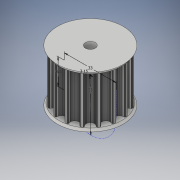
# Autodesk Inventor part: 8M_pulley_39mm
Saved by Autodesk Inventor 2019 (Build 230136000, 136)
## iProperties
Created: 2019-09-25
Part Number: 8M_pulley_39mm
Material: Generic
Document SubType Name: Modeling
Designer: isaac
Density: 1 g/cm^3
Appearance: Default
Author: isaac
Autodesk Inventor part; units mm, degrees
(part 1 of 2)
sketch "Sketch1" plane through (0, 0, 0) normal (0, 1, 0) x (-1, 0, 0)
  line L0 (-19.3836, -3.3292) -> (-19.3679, -3.8461)
  line L1 (-19.3679, -3.8461) -> (-19.3017, -4.359)
  line L2 (-19.3017, -4.359) -> (-19.3017, -4.3591)
  line L3 (-19.3017, -4.3591) -> (-19.2707, -4.4187)
  line L4 (-19.2707, -4.4187) -> (-19.1879, -4.5272)
  line L5 (-19.1879, -4.5272) -> (-19.0895, -4.6186)
  line L6 (-19.0895, -4.6186) -> (-18.9784, -4.6913)
  line L7 (-18.9784, -4.6913) -> (-18.8571, -4.7439)
  line L8 (-18.8571, -4.7439) -> (-18.7285, -4.775)
  line L9 (-18.7285, -4.775) -> (-18.5953, -4.7829)
  line L10 (-18.5953, -4.7829) -> (-18.4601, -4.7664)
  line L11 (-18.4601, -4.7664) -> (-17.6457, -4.5321)
  line L12 (-17.6457, -4.5321) -> (-17.4212, -4.494)
  line L13 (-17.4212, -4.494) -> (-17.1971, -4.4763)
  line L14 (-17.1971, -4.4763) -> (-16.9744, -4.4785)
  line L15 (-16.9744, -4.4785) -> (-16.7542, -4.4999)
  line L16 (-16.7542, -4.4999) -> (-16.5375, -4.5401)
  line L17 (-16.5375, -4.5401) -> (-16.3256, -4.5984)
  line L18 (-16.3256, -4.5984) -> (-16.1194, -4.6743)
  line L19 (-16.1194, -4.6743) -> (-15.92, -4.7673)
  line L20 (-15.92, -4.7673) -> (-15.7285, -4.8767)
  line L21 (-15.7285, -4.8767) -> (-15.5461, -5.0021)
  line L22 (-15.5461, -5.0021) -> (-15.3737, -5.1428)
  line L23 (-15.3737, -5.1428) -> (-15.2125, -5.2982)
  line L24 (-15.2125, -5.2982) -> (-15.0635, -5.4679)
  line L25 (-15.0635, -5.4679) -> (-14.9279, -5.6513)
  line L26 (-14.9279, -5.6513) -> (-14.8067, -5.8478)
  line L27 (-14.8067, -5.8478) -> (-14.7009, -6.0568)
  line L28 (-14.7009, -6.0568) -> (-14.6281, -6.2792)
  line L29 (-14.6281, -6.2792) -> (-14.575, -6.5038)
  line L30 (-14.575, -6.5038) -> (-14.5414, -6.7293)
  line L31 (-14.5414, -6.7293) -> (-14.5268, -6.9545)
  line L32 (-14.5268, -6.9545) -> (-14.5309, -7.1784)
  line L33 (-14.5309, -7.1784) -> (-14.5534, -7.3996)
  line L34 (-14.5534, -7.3996) -> (-14.5938, -7.6172)
  line L35 (-14.5938, -7.6172) -> (-14.6518, -7.8299)
  line L36 (-14.6518, -7.8299) -> (-14.7271, -8.0366)
  line L37 (-14.7271, -8.0366) -> (-14.8192, -8.2361)
  line L38 (-14.8192, -8.2361) -> (-14.9278, -8.4272)
  line L39 (-14.9278, -8.4272) -> (-15.0525, -8.6088)
  line L40 (-15.0525, -8.6088) -> (-15.193, -8.7797)
  line L41 (-15.193, -8.7797) -> (-15.3488, -8.9388)
  line L42 (-15.3488, -8.9388) -> (-15.5197, -9.0849)
  line L43 (-15.5197, -9.0849) -> (-15.7052, -9.2168)
  line L44 (-15.7052, -9.2168) -> (-16.4468, -9.627)
  line L45 (-16.4468, -9.627) -> (-16.554, -9.711)
  line L46 (-16.554, -9.711) -> (-16.6426, -9.8109)
  line L47 (-16.6426, -9.8109) -> (-16.7116, -9.9238)
  line L48 (-16.7116, -9.9238) -> (-16.7601, -10.0467)
  line L49 (-16.7601, -10.0467) -> (-16.7873, -10.1767)
  line L50 (-16.7873, -10.1767) -> (-16.7923, -10.3108)
  line L51 (-16.7923, -10.3108) -> (-16.7741, -10.4461)
  line L52 (-16.7741, -10.4461) -> (-16.7538, -10.5101)
  line L53 (-16.7538, -10.5101) -> (-16.7538, -10.5102)
  line L54 (-16.7538, -10.5102) -> (-16.4879, -10.9538)
  line L55 (-16.4879, -10.9538) -> (-16.1799, -11.3692)
  line L56 (-16.1799, -11.3692) -> (-16.1653, -11.3814)
  line L57 (-16.1653, -11.3814) -> (-16.1652, -11.3814)
  line L58 (-16.1652, -11.3814) -> (-16.1284, -11.4124)
  line L59 (-16.1284, -11.4124) -> (-16.0103, -11.481)
  line L60 (-16.0103, -11.481) -> (-15.8845, -11.5278)
  line L61 (-15.8845, -11.5278) -> (-15.754, -11.5524)
  line L62 (-15.754, -11.5524) -> (-15.6218, -11.5546)
  line L63 (-15.6218, -11.5546) -> (-15.4911, -11.5341)
  line L64 (-15.4911, -11.5341) -> (-15.365, -11.4905)
  line L65 (-15.365, -11.4905) -> (-15.2464, -11.4235)
  line L66 (-15.2464, -11.4235) -> (-14.5837, -10.8953)
  line L67 (-14.5837, -10.8953) -> (-14.3909, -10.7742)
  line L68 (-14.3909, -10.7742) -> (-14.1905, -10.6721)
  line L69 (-14.1905, -10.6721) -> (-13.984, -10.5889)
  line L70 (-13.984, -10.5889) -> (-13.7723, -10.5244)
  line L71 (-13.7723, -10.5244) -> (-13.5568, -10.4787)
  line L72 (-13.5568, -10.4787) -> (-13.3387, -10.4514)
  line L73 (-13.3387, -10.4514) -> (-13.1191, -10.4426)
  line L74 (-13.1191, -10.4426) -> (-12.8993, -10.4522)
  line L75 (-12.8993, -10.4522) -> (-12.6806, -10.4801)
  line L76 (-12.6806, -10.4801) -> (-12.464, -10.526)
  line L77 (-12.464, -10.526) -> (-12.2509, -10.5901)
  line L78 (-12.2509, -10.5901) -> (-12.0425, -10.672)
  line L79 (-12.0425, -10.672) -> (-11.8399, -10.7718)
  line L80 (-11.8399, -10.7718) -> (-11.6444, -10.8893)
  line L81 (-11.6444, -10.8893) -> (-11.4572, -11.0244)
  line L82 (-11.4572, -11.0244) -> (-11.2796, -11.177)
  line L83 (-11.2796, -11.177) -> (-11.1271, -11.3547)
  line L84 (-11.1271, -11.3547) -> (-10.9922, -11.5418)
  line L85 (-10.9922, -11.5418) -> (-10.8748, -11.7373)
  line L86 (-10.8748, -11.7373) -> (-10.7752, -11.9398)
  line L87 (-10.7752, -11.9398) -> (-10.6933, -12.1481)
  line L88 (-10.6933, -12.1481) -> (-10.6293, -12.3611)
  line L89 (-10.6293, -12.3611) -> (-10.5834, -12.5776)
  line L90 (-10.5834, -12.5776) -> (-10.5556, -12.7963)
  line L91 (-10.5556, -12.7963) -> (-10.546, -13.0161)
  line L92 (-10.546, -13.0161) -> (-10.5548, -13.2356)
  line L93 (-10.5548, -13.2356) -> (-10.582, -13.4537)
  line L94 (-10.582, -13.4537) -> (-10.6278, -13.6692)
  line L95 (-10.6278, -13.6692) -> (-10.6921, -13.8809)
  line L96 (-10.6921, -13.8809) -> (-10.7753, -14.0875)
  line L97 (-10.7753, -14.0875) -> (-10.8772, -14.2879)
  line L98 (-10.8772, -14.2879) -> (-10.9981, -14.4808)
  line L99 (-10.9981, -14.4808) -> (-11.5263, -15.1435)
  line L100 (-11.5263, -15.1435) -> (-11.5932, -15.2621)
  line L101 (-11.5932, -15.2621) -> (-11.6368, -15.3883)
  line L102 (-11.6368, -15.3883) -> (-11.6573, -15.519)
  line L103 (-11.6573, -15.519) -> (-11.6551, -15.6512)
  line L104 (-11.6551, -15.6512) -> (-11.6305, -15.7817)
  line L105 (-11.6305, -15.7817) -> (-11.5838, -15.9075)
  line L106 (-11.5838, -15.9075) -> (-11.5152, -16.0255)
  line L107 (-11.5152, -16.0255) -> (-11.472, -16.0769)
  line L108 (-11.472, -16.0769) -> (-11.472, -16.077)
  line L109 (-11.472, -16.077) -> (-11.0566, -16.385)
  line L110 (-11.0566, -16.385) -> (-10.613, -16.6509)
  line L111 (-10.613, -16.6509) -> (-10.5948, -16.6567)
  line L112 (-10.5948, -16.6567) -> (-10.5489, -16.6712)
  line L113 (-10.5489, -16.6712) -> (-10.4136, -16.6894)
  line L114 (-10.4136, -16.6894) -> (-10.2794, -16.6844)
  line L115 (-10.2794, -16.6844) -> (-10.1494, -16.6572)
  line L116 (-10.1494, -16.6572) -> (-10.0264, -16.6087)
  line L117 (-10.0264, -16.6087) -> (-9.9135, -16.5397)
  line L118 (-9.9135, -16.5397) -> (-9.8137, -16.4511)
  line L119 (-9.8137, -16.4511) -> (-9.7298, -16.3439)
  line L120 (-9.7298, -16.3439) -> (-9.3196, -15.6022)
  line L121 (-9.3196, -15.6022) -> (-9.1879, -15.4166)
  line L122 (-9.1879, -15.4166) -> (-9.0419, -15.2456)
  line L123 (-9.0419, -15.2456) -> (-8.8829, -15.0896)
  line L124 (-8.8829, -15.0896) -> (-8.7121, -14.9491)
  line L125 (-8.7121, -14.9491) -> (-8.5305, -14.8243)
  line L126 (-8.5305, -14.8243) -> (-8.3394, -14.7156)
  line L127 (-8.3394, -14.7156) -> (-8.1399, -14.6235)
  line L128 (-8.1399, -14.6235) -> (-7.9332, -14.5482)
  line L129 (-7.9332, -14.5482) -> (-7.7204, -14.4902)
  line L130 (-7.7204, -14.4902) -> (-7.5028, -14.4498)
  line L131 (-7.5028, -14.4498) -> (-7.2814, -14.4274)
  line L132 (-7.2814, -14.4274) -> (-7.0575, -14.4233)
  line L133 (-7.0575, -14.4233) -> (-6.8321, -14.438)
  line L134 (-6.8321, -14.438) -> (-6.6066, -14.4717)
  line L135 (-6.6066, -14.4717) -> (-6.3819, -14.5249)
  line L136 (-6.3819, -14.5249) -> (-6.1594, -14.598)
  line L137 (-6.1594, -14.598) -> (-5.9505, -14.7037)
  line L138 (-5.9505, -14.7037) -> (-5.7542, -14.825)
  line L139 (-5.7542, -14.825) -> (-5.571, -14.9607)
  line L140 (-5.571, -14.9607) -> (-5.4014, -15.1096)
  line L141 (-5.4014, -15.1096) -> (-5.2461, -15.2708)
  line L142 (-5.2461, -15.2708) -> (-5.1055, -15.4432)
  line L143 (-5.1055, -15.4432) -> (-4.9802, -15.6256)
  line L144 (-4.9802, -15.6256) -> (-4.8708, -15.8171)
  line L145 (-4.8708, -15.8171) -> (-4.7779, -16.0164)
  line L146 (-4.7779, -16.0164) -> (-4.702, -16.2226)
  line L147 (-4.702, -16.2226) -> (-4.6437, -16.4345)
  line L148 (-4.6437, -16.4345) -> (-4.6034, -16.6511)
  line L149 (-4.6034, -16.6511) -> (-4.5819, -16.8713)
  line L150 (-4.5819, -16.8713) -> (-4.5796, -17.094)
  line L151 (-4.5796, -17.094) -> (-4.5971, -17.3181)
  line L152 (-4.5971, -17.3181) -> (-4.635, -17.5426)
  line L153 (-4.635, -17.5426) -> (-4.8693, -18.357)
  line L154 (-4.8693, -18.357) -> (-4.8858, -18.4922)
  line L155 (-4.8858, -18.4922) -> (-4.8777, -18.6255)
  line L156 (-4.8777, -18.6255) -> (-4.8467, -18.7541)
  line L157 (-4.8467, -18.7541) -> (-4.7941, -18.8753)
  line L158 (-4.7941, -18.8753) -> (-4.7214, -18.9865)
  line L159 (-4.7214, -18.9865) -> (-4.6301, -19.0848)
  line L160 (-4.6301, -19.0848) -> (-4.5216, -19.1676)
  line L161 (-4.5216, -19.1676) -> (-4.5047, -19.1764)
  line L162 (-4.5047, -19.1764) -> (-4.462, -19.1986)
  line L163 (-4.462, -19.1986) -> (-4.462, -19.1986)
  line L164 (-4.462, -19.1986) -> (-3.9603, -19.3243)
  line L165 (-3.9603, -19.3243) -> (-3.4487, -19.4002)
  line L166 (-3.4487, -19.4002) -> (-3.4297, -19.3986)
  line L167 (-3.4297, -19.3986) -> (-3.4297, -19.3986)
  line L168 (-3.4297, -19.3986) -> (-3.3817, -19.3944)
  line L169 (-3.3817, -19.3944) -> (-3.2498, -19.3594)
  line L170 (-3.2498, -19.3594) -> (-3.1277, -19.3035)
  line L171 (-3.1277, -19.3035) -> (-3.018, -19.2286)
  line L172 (-3.018, -19.2286) -> (-2.923, -19.1367)
  line L173 (-2.923, -19.1367) -> (-2.8451, -19.0298)
  line L174 (-2.8451, -19.0298) -> (-2.7867, -18.9097)
  line L175 (-2.7867, -18.9097) -> (-2.7503, -18.7785)
  line L176 (-2.7503, -18.7785) -> (-2.655, -17.9364)
  line L177 (-2.655, -17.9364) -> (-2.6043, -17.7145)
  line L178 (-2.6043, -17.7145) -> (-2.5349, -17.5006)
  line L179 (-2.5349, -17.5006) -> (-2.4477, -17.2957)
  line L180 (-2.4477, -17.2957) -> (-2.3436, -17.1005)
  line L181 (-2.3436, -17.1005) -> (-2.2236, -16.9157)
  line L182 (-2.2236, -16.9157) -> (-2.0886, -16.7422)
  line L183 (-2.0886, -16.7422) -> (-1.9395, -16.5807)
  line L184 (-1.9395, -16.5807) -> (-1.7773, -16.4322)
  line L185 (-1.7773, -16.4322) -> (-1.603, -16.2972)
  line L186 (-1.603, -16.2972) -> (-1.4173, -16.1766)
  line L187 (-1.4173, -16.1766) -> (-1.2214, -16.0712)
  line L188 (-1.2214, -16.0712) -> (-1.016, -15.9817)
  line L189 (-1.016, -15.9817) -> (-0.8022, -15.909)
  line L190 (-0.8022, -15.909) -> (-0.5809, -15.8539)
  line L191 (-0.5809, -15.8539) -> (-0.353, -15.8171)
  line L192 (-0.353, -15.8171) -> (-0.1195, -15.7994)
  line L193 (-0.1195, -15.7994) -> (0.1139, -15.8172)
  line L194 (0.1139, -15.8172) -> (0.3417, -15.8541)
  line L195 (0.3417, -15.8541) -> (0.5629, -15.9093)
  line L196 (0.5629, -15.9093) -> (0.7766, -15.9821)
  line L197 (0.7766, -15.9821) -> (0.9818, -16.0715)
  line L198 (0.9818, -16.0715) -> (1.1776, -16.1769)
  line L199 (1.1776, -16.1769) -> (1.3632, -16.2975)
  line L200 (1.3632, -16.2975) -> (1.5376, -16.4325)
  line L201 (1.5376, -16.4325) -> (1.6997, -16.581)
  line L202 (1.6997, -16.581) -> (1.8488, -16.7424)
  line L203 (1.8488, -16.7424) -> (1.9838, -16.9159)
  line L204 (1.9838, -16.9159) -> (2.1039, -17.1006)
  line L205 (2.1039, -17.1006) -> (2.208, -17.2958)
  line L206 (2.208, -17.2958) -> (2.2954, -17.5007)
  line L207 (2.2954, -17.5007) -> (2.3649, -17.7144)
  line L208 (2.3649, -17.7144) -> (2.4158, -17.9363)
  line L209 (2.4158, -17.9363) -> (2.511, -18.7784)
  line L210 (2.511, -18.7784) -> (2.5476, -18.9096)
  line L211 (2.5476, -18.9096) -> (2.606, -19.0297)
  line L212 (2.606, -19.0297) -> (2.6839, -19.1366)
  line L213 (2.6839, -19.1366) -> (2.7789, -19.2285)
  line L214 (2.7789, -19.2285) -> (2.8886, -19.3034)
  line L215 (2.8886, -19.3034) -> (3.0106, -19.3593)
  line L216 (3.0106, -19.3593) -> (3.1425, -19.3943)
  line L217 (3.1425, -19.3943) -> (3.1615, -19.3959)
  line L218 (3.1615, -19.3959) -> (3.2094, -19.4001)
  line L219 (3.2094, -19.4001) -> (3.2095, -19.4001)
  line L220 (3.2095, -19.4001) -> (3.7264, -19.3845)
  line L221 (3.7264, -19.3845) -> (4.2393, -19.3182)
  line L222 (4.2393, -19.3182) -> (4.2562, -19.3094)
  line L223 (4.2562, -19.3094) -> (4.2563, -19.3094)
  line L224 (4.2563, -19.3094) -> (4.299, -19.2872)
  line L225 (4.299, -19.2872) -> (4.4075, -19.2044)
  line L226 (4.4075, -19.2044) -> (4.4989, -19.106)
  line L227 (4.4989, -19.106) -> (4.5716, -18.9949)
  line L228 (4.5716, -18.9949) -> (4.6242, -18.8736)
  line L229 (4.6242, -18.8736) -> (4.6553, -18.745)
  line L230 (4.6553, -18.745) -> (4.6632, -18.6118)
  line L231 (4.6632, -18.6118) -> (4.6467, -18.4766)
  line L232 (4.6467, -18.4766) -> (4.4124, -17.6622)
  line L233 (4.4124, -17.6622) -> (4.3743, -17.4377)
  line L234 (4.3743, -17.4377) -> (4.3566, -17.2136)
  line L235 (4.3566, -17.2136) -> (4.3588, -16.9909)
  line L236 (4.3588, -16.9909) -> (4.3802, -16.7707)
  line L237 (4.3802, -16.7707) -> (4.4204, -16.554)
  line L238 (4.4204, -16.554) -> (4.4787, -16.3421)
  line L239 (4.4787, -16.3421) -> (4.5546, -16.1359)
  line L240 (4.5546, -16.1359) -> (4.6476, -15.9365)
  line L241 (4.6476, -15.9365) -> (4.757, -15.745)
  line L242 (4.757, -15.745) -> (4.8824, -15.5626)
  line L243 (4.8824, -15.5626) -> (5.0231, -15.3902)
  line L244 (5.0231, -15.3902) -> (5.1785, -15.229)
  line L245 (5.1785, -15.229) -> (5.3483, -15.08)
  line L246 (5.3483, -15.08) -> (5.5316, -14.9444)
  line L247 (5.5316, -14.9444) -> (5.7281, -14.8232)
  line L248 (5.7281, -14.8232) -> (5.9371, -14.7174)
  line L249 (5.9371, -14.7174) -> (6.1595, -14.6446)
  line L250 (6.1595, -14.6446) -> (6.3841, -14.5915)
  line L251 (6.3841, -14.5915) -> (6.6096, -14.5579)
  line L252 (6.6096, -14.5579) -> (6.8348, -14.5433)
  line L253 (6.8348, -14.5433) -> (7.0587, -14.5474)
  line L254 (7.0587, -14.5474) -> (7.28, -14.5699)
  line L255 (7.28, -14.5699) -> (7.4975, -14.6103)
  line L256 (7.4975, -14.6103) -> (7.7102, -14.6683)
  line L257 (7.7102, -14.6683) -> (7.9169, -14.7436)
  line L258 (7.9169, -14.7436) -> (8.1164, -14.8357)
  line L259 (8.1164, -14.8357) -> (8.3075, -14.9443)
  line L260 (8.3075, -14.9443) -> (8.4891, -15.069)
  line L261 (8.4891, -15.069) -> (8.66, -15.2095)
  line L262 (8.66, -15.2095) -> (8.8191, -15.3653)
  line L263 (8.8191, -15.3653) -> (8.9652, -15.5362)
  line L264 (8.9652, -15.5362) -> (9.0971, -15.7217)
  line L265 (9.0971, -15.7217) -> (9.5073, -16.4633)
  line L266 (9.5073, -16.4633) -> (9.5913, -16.5705)
  line L267 (9.5913, -16.5705) -> (9.6912, -16.6591)
  line L268 (9.6912, -16.6591) -> (9.8041, -16.7281)
  line L269 (9.8041, -16.7281) -> (9.927, -16.7766)
  line L270 (9.927, -16.7766) -> (10.057, -16.8038)
  line L271 (10.057, -16.8038) -> (10.1911, -16.8088)
  line L272 (10.1911, -16.8088) -> (10.3264, -16.7906)
  line L273 (10.3264, -16.7906) -> (10.3446, -16.7848)
  line L274 (10.3446, -16.7848) -> (10.3904, -16.7703)
  line L275 (10.3904, -16.7703) -> (10.3905, -16.7703)
  line L276 (10.3905, -16.7703) -> (10.8341, -16.5044)
  line L277 (10.8341, -16.5044) -> (11.2495, -16.1964)
  line L278 (11.2495, -16.1964) -> (11.2495, -16.1963)
  line L279 (11.2495, -16.1963) -> (11.2927, -16.1449)
  line L280 (11.2927, -16.1449) -> (11.3613, -16.0268)
  line L281 (11.3613, -16.0268) -> (11.4081, -15.901)
  line L282 (11.4081, -15.901) -> (11.4327, -15.7705)
  line L283 (11.4327, -15.7705) -> (11.4349, -15.6383)
  line L284 (11.4349, -15.6383) -> (11.4144, -15.5076)
  line L285 (11.4144, -15.5076) -> (11.3708, -15.3815)
  line L286 (11.3708, -15.3815) -> (11.3038, -15.2629)
  line L287 (11.3038, -15.2629) -> (10.7756, -14.6002)
  line L288 (10.7756, -14.6002) -> (10.6545, -14.4074)
  line L289 (10.6545, -14.4074) -> (10.5524, -14.207)
  line L290 (10.5524, -14.207) -> (10.4692, -14.0005)
  line L291 (10.4692, -14.0005) -> (10.4047, -13.7888)
  line L292 (10.4047, -13.7888) -> (10.359, -13.5733)
  line L293 (10.359, -13.5733) -> (10.3317, -13.3552)
  line L294 (10.3317, -13.3552) -> (10.3229, -13.1356)
  line L295 (10.3229, -13.1356) -> (10.3325, -12.9158)
  line L296 (10.3325, -12.9158) -> (10.3604, -12.6971)
  line L297 (10.3604, -12.6971) -> (10.4063, -12.4805)
  line L298 (10.4063, -12.4805) -> (10.4704, -12.2674)
  line L299 (10.4704, -12.2674) -> (10.5523, -12.059)
  line L300 (10.5523, -12.059) -> (10.6521, -11.8564)
  line L301 (10.6521, -11.8564) -> (10.7696, -11.6609)
  line L302 (10.7696, -11.6609) -> (10.9047, -11.4737)
  line L303 (10.9047, -11.4737) -> (11.0573, -11.2961)
  line L304 (11.0573, -11.2961) -> (11.235, -11.1436)
  line L305 (11.235, -11.1436) -> (11.4221, -11.0087)
  line L306 (11.4221, -11.0087) -> (11.6176, -10.8913)
  line L307 (11.6176, -10.8913) -> (11.8201, -10.7917)
  line L308 (11.8201, -10.7917) -> (12.0285, -10.7098)
  line L309 (12.0285, -10.7098) -> (12.2414, -10.6459)
  line L310 (12.2414, -10.6459) -> (12.4579, -10.6)
  line L311 (12.4579, -10.6) -> (12.6766, -10.5722)
  line L312 (12.6766, -10.5722) -> (12.8964, -10.5626)
  line L313 (12.8964, -10.5626) -> (13.1159, -10.5713)
  line L314 (13.1159, -10.5713) -> (13.334, -10.5985)
  line L315 (13.334, -10.5985) -> (13.5495, -10.6443)
  line L316 (13.5495, -10.6443) -> (13.7612, -10.7086)
  line L317 (13.7612, -10.7086) -> (13.9678, -10.7918)
  line L318 (13.9678, -10.7918) -> (14.1682, -10.8937)
  line L319 (14.1682, -10.8937) -> (14.3611, -11.0146)
  line L320 (14.3611, -11.0146) -> (15.0238, -11.5428)
  line L321 (15.0238, -11.5428) -> (15.1424, -11.6097)
  line L322 (15.1424, -11.6097) -> (15.2686, -11.6533)
  line L323 (15.2686, -11.6533) -> (15.3993, -11.6738)
  line L324 (15.3993, -11.6738) -> (15.5315, -11.6716)
  line L325 (15.5315, -11.6716) -> (15.662, -11.647)
  line L326 (15.662, -11.647) -> (15.7878, -11.6003)
  line L327 (15.7878, -11.6003) -> (15.9058, -11.5317)
  line L328 (15.9058, -11.5317) -> (15.9204, -11.5195)
  line L329 (15.9204, -11.5195) -> (15.9572, -11.4885)
  line L330 (15.9572, -11.4885) -> (15.9574, -11.4885)
  line L331 (15.9574, -11.4885) -> (16.2654, -11.0731)
  line L332 (16.2654, -11.0731) -> (16.5313, -10.6295)
  line L333 (16.5313, -10.6295) -> (16.5313, -10.6294)
  line L334 (16.5313, -10.6294) -> (16.5516, -10.5654)
  line L335 (16.5516, -10.5654) -> (16.5697, -10.4301)
  line L336 (16.5697, -10.4301) -> (16.5647, -10.2959)
  line L337 (16.5647, -10.2959) -> (16.5375, -10.1659)
  line L338 (16.5375, -10.1659) -> (16.489, -10.0429)
  line L339 (16.489, -10.0429) -> (16.42, -9.9301)
  line L340 (16.42, -9.9301) -> (16.3314, -9.8302)
  line L341 (16.3314, -9.8302) -> (16.2242, -9.7463)
  line L342 (16.2242, -9.7463) -> (15.4826, -9.3362)
  line L343 (15.4826, -9.3362) -> (15.297, -9.2044)
  line L344 (15.297, -9.2044) -> (15.1259, -9.0584)
  line L345 (15.1259, -9.0584) -> (14.9699, -8.8994)
  line L346 (14.9699, -8.8994) -> (14.8294, -8.7286)
  line L347 (14.8294, -8.7286) -> (14.7046, -8.547)
  line L348 (14.7046, -8.547) -> (14.5959, -8.3559)
  line L349 (14.5959, -8.3559) -> (14.5038, -8.1564)
  line L350 (14.5038, -8.1564) -> (14.4286, -7.9497)
  line L351 (14.4286, -7.9497) -> (14.3705, -7.7369)
  line L352 (14.3705, -7.7369) -> (14.3301, -7.5193)
  line L353 (14.3301, -7.5193) -> (14.3077, -7.2979)
  line L354 (14.3077, -7.2979) -> (14.3036, -7.074)
  line L355 (14.3036, -7.074) -> (14.3183, -6.8486)
  line L356 (14.3183, -6.8486) -> (14.352, -6.6231)
  line L357 (14.352, -6.6231) -> (14.4052, -6.3984)
  line L358 (14.4052, -6.3984) -> (14.4783, -6.1759)
  line L359 (14.4783, -6.1759) -> (14.584, -5.9671)
  line L360 (14.584, -5.9671) -> (14.7053, -5.7708)
  line L361 (14.7053, -5.7708) -> (14.841, -5.5875)
  line L362 (14.841, -5.5875) -> (14.9899, -5.418)
  line L363 (14.9899, -5.418) -> (15.1511, -5.2626)
  line L364 (15.1511, -5.2626) -> (15.3235, -5.122)
  line L365 (15.3235, -5.122) -> (15.5059, -4.9967)
  line L366 (15.5059, -4.9967) -> (15.6974, -4.8874)
  line L367 (15.6974, -4.8874) -> (15.8967, -4.7944)
  line L368 (15.8967, -4.7944) -> (16.1029, -4.7185)
  line L369 (16.1029, -4.7185) -> (16.3148, -4.6602)
  line L370 (16.3148, -4.6602) -> (16.5314, -4.62)
  line L371 (16.5314, -4.62) -> (16.7516, -4.5984)
  line L372 (16.7516, -4.5984) -> (16.9743, -4.5961)
  line L373 (16.9743, -4.5961) -> (17.1984, -4.6137)
  line L374 (17.1984, -4.6137) -> (17.4229, -4.6516)
  line L375 (17.4229, -4.6516) -> (18.2373, -4.8858)
  line L376 (18.2373, -4.8858) -> (18.3725, -4.9023)
  line L377 (18.3725, -4.9023) -> (18.5058, -4.8943)
  line L378 (18.5058, -4.8943) -> (18.6344, -4.8632)
  line L379 (18.6344, -4.8632) -> (18.7556, -4.8107)
  line L380 (18.7556, -4.8107) -> (18.8668, -4.738)
  line L381 (18.8668, -4.738) -> (18.9651, -4.6466)
  line L382 (18.9651, -4.6466) -> (19.0479, -4.5381)
  line L383 (19.0479, -4.5381) -> (19.0789, -4.4785)
  line L384 (19.0789, -4.4785) -> (19.0789, -4.4785)
  line L385 (19.0789, -4.4785) -> (19.2046, -3.9768)
  line L386 (19.2046, -3.9768) -> (19.2805, -3.4652)
  line L387 (19.2805, -3.4652) -> (19.2805, -3.4652)
  line L388 (19.2805, -3.4652) -> (19.2747, -3.3982)
  line L389 (19.2747, -3.3982) -> (19.2397, -3.2663)
  line L390 (19.2397, -3.2663) -> (19.1838, -3.1442)
  line L391 (19.1838, -3.1442) -> (19.1089, -3.0345)
  line L392 (19.1089, -3.0345) -> (19.017, -2.9395)
  line L393 (19.017, -2.9395) -> (18.9101, -2.8616)
  line L394 (18.9101, -2.8616) -> (18.79, -2.8032)
  line L395 (18.79, -2.8032) -> (18.6588, -2.7668)
  line L396 (18.6588, -2.7668) -> (17.8167, -2.6716)
  line L397 (17.8167, -2.6716) -> (17.5948, -2.6209)
  line L398 (17.5948, -2.6209) -> (17.3809, -2.5514)
  line L399 (17.3809, -2.5514) -> (17.176, -2.4642)
  line L400 (17.176, -2.4642) -> (16.9809, -2.3601)
  line L401 (16.9809, -2.3601) -> (16.7961, -2.2401)
  line L402 (16.7961, -2.2401) -> (16.6226, -2.1051)
  line L403 (16.6226, -2.1051) -> (16.4611, -1.956)
  line L404 (16.4611, -1.956) -> (16.3125, -1.7938)
  line L405 (16.3125, -1.7938) -> (16.1775, -1.6195)
  line L406 (16.1775, -1.6195) -> (16.0569, -1.4338)
  line L407 (16.0569, -1.4338) -> (15.9515, -1.2379)
  line L408 (15.9515, -1.2379) -> (15.862, -1.0326)
  line L409 (15.862, -1.0326) -> (15.7893, -0.8188)
  line L410 (15.7893, -0.8188) -> (15.7342, -0.5974)
  line L411 (15.7342, -0.5974) -> (15.6974, -0.3695)
  line L412 (15.6974, -0.3695) -> (15.6797, -0.136)
  line L413 (15.6797, -0.136) -> (15.6975, 0.0974)
  line L414 (15.6975, 0.0974) -> (15.7344, 0.3252)
  line L415 (15.7344, 0.3252) -> (15.7896, 0.5464)
  line L416 (15.7896, 0.5464) -> (15.8624, 0.76)
  line L417 (15.8624, 0.76) -> (15.9518, 0.9653)
  line L418 (15.9518, 0.9653) -> (16.0572, 1.1611)
  line L419 (16.0572, 1.1611) -> (16.1778, 1.3467)
  line L420 (16.1778, 1.3467) -> (16.3128, 1.521)
  line L421 (16.3128, 1.521) -> (16.4613, 1.6832)
  line L422 (16.4613, 1.6832) -> (16.6227, 1.8323)
  line L423 (16.6227, 1.8323) -> (16.7962, 1.9673)
  line L424 (16.7962, 1.9673) -> (16.9809, 2.0873)
  line L425 (16.9809, 2.0873) -> (17.1761, 2.1915)
  line L426 (17.1761, 2.1915) -> (17.381, 2.2788)
  line L427 (17.381, 2.2788) -> (17.5947, 2.3484)
  line L428 (17.5947, 2.3484) -> (17.8166, 2.3993)
  line L429 (17.8166, 2.3993) -> (18.6587, 2.4945)
  line L430 (18.6587, 2.4945) -> (18.7899, 2.5311)
  line L431 (18.7899, 2.5311) -> (18.91, 2.5895)
  line L432 (18.91, 2.5895) -> (19.0169, 2.6674)
  line L433 (19.0169, 2.6674) -> (19.1088, 2.7623)
  line L434 (19.1088, 2.7623) -> (19.1837, 2.872)
  line L435 (19.1837, 2.872) -> (19.2396, 2.994)
  line L436 (19.2396, 2.994) -> (19.2746, 3.126)
  line L437 (19.2746, 3.126) -> (19.2804, 3.1929)
  line L438 (19.2804, 3.1929) -> (19.2804, 3.1929)
  line L439 (19.2804, 3.1929) -> (19.2648, 3.7099)
  line L440 (19.2648, 3.7099) -> (19.1986, 4.2228)
  line L441 (19.1986, 4.2228) -> (19.1986, 4.2229)
  line L442 (19.1986, 4.2229) -> (19.1676, 4.2825)
  line L443 (19.1676, 4.2825) -> (19.0848, 4.391)
  line L444 (19.0848, 4.391) -> (18.9864, 4.4824)
  line L445 (18.9864, 4.4824) -> (18.8753, 4.5551)
  line L446 (18.8753, 4.5551) -> (18.754, 4.6077)
  line L447 (18.754, 4.6077) -> (18.6254, 4.6387)
  line L448 (18.6254, 4.6387) -> (18.4922, 4.6467)
  line L449 (18.4922, 4.6467) -> (18.357, 4.6302)
  line L450 (18.357, 4.6302) -> (17.5426, 4.3959)
  line L451 (17.5426, 4.3959) -> (17.3181, 4.3578)
  line L452 (17.3181, 4.3578) -> (17.094, 4.3401)
  line L453 (17.094, 4.3401) -> (16.8713, 4.3423)
  line L454 (16.8713, 4.3423) -> (16.6511, 4.3637)
  line L455 (16.6511, 4.3637) -> (16.4344, 4.4039)
  line L456 (16.4344, 4.4039) -> (16.2225, 4.4622)
  line L457 (16.2225, 4.4622) -> (16.0163, 4.5381)
  line L458 (16.0163, 4.5381) -> (15.8169, 4.6311)
  line L459 (15.8169, 4.6311) -> (15.6254, 4.7405)
  line L460 (15.6254, 4.7405) -> (15.443, 4.8659)
  line L461 (15.443, 4.8659) -> (15.2706, 5.0065)
  line L462 (15.2706, 5.0065) -> (15.1094, 5.162)
  line L463 (15.1094, 5.162) -> (14.9604, 5.3317)
  line L464 (14.9604, 5.3317) -> (14.8248, 5.5151)
  line L465 (14.8248, 5.5151) -> (14.7036, 5.7116)
  line L466 (14.7036, 5.7116) -> (14.5978, 5.9206)
  line L467 (14.5978, 5.9206) -> (14.525, 6.143)
  line L468 (14.525, 6.143) -> (14.4719, 6.3676)
  line L469 (14.4719, 6.3676) -> (14.4383, 6.593)
  line L470 (14.4383, 6.593) -> (14.4237, 6.8183)
  line L471 (14.4237, 6.8183) -> (14.4278, 7.0421)
  line L472 (14.4278, 7.0421) -> (14.4503, 7.2634)
  line L473 (14.4503, 7.2634) -> (14.4907, 7.481)
  line L474 (14.4907, 7.481) -> (14.5487, 7.6937)
  line L475 (14.5487, 7.6937) -> (14.624, 7.9004)
  line L476 (14.624, 7.9004) -> (14.7161, 8.0999)
  line L477 (14.7161, 8.0999) -> (14.8247, 8.291)
  line L478 (14.8247, 8.291) -> (14.9494, 8.4726)
  line L479 (14.9494, 8.4726) -> (15.0899, 8.6435)
  line L480 (15.0899, 8.6435) -> (15.2457, 8.8026)
  line L481 (15.2457, 8.8026) -> (15.4166, 8.9487)
  line L482 (15.4166, 8.9487) -> (15.6021, 9.0806)
  line L483 (15.6021, 9.0806) -> (16.3437, 9.4908)
  line L484 (16.3437, 9.4908) -> (16.4509, 9.5748)
  line L485 (16.4509, 9.5748) -> (16.5395, 9.6747)
  line L486 (16.5395, 9.6747) -> (16.6085, 9.7876)
  line L487 (16.6085, 9.7876) -> (16.657, 9.9105)
  line L488 (16.657, 9.9105) -> (16.6842, 10.0405)
  line L489 (16.6842, 10.0405) -> (16.6892, 10.1746)
  line L490 (16.6892, 10.1746) -> (16.671, 10.3099)
  line L491 (16.671, 10.3099) -> (16.6507, 10.3739)
  line L492 (16.6507, 10.3739) -> (16.6507, 10.374)
  line L493 (16.6507, 10.374) -> (16.3848, 10.8176)
  line L494 (16.3848, 10.8176) -> (16.0768, 11.233)
  line L495 (16.0768, 11.233) -> (16.0622, 11.2452)
  line L496 (16.0622, 11.2452) -> (16.0621, 11.2452)
  line L497 (16.0621, 11.2452) -> (16.0253, 11.2762)
  line L498 (16.0253, 11.2762) -> (15.9072, 11.3448)
  line L499 (15.9072, 11.3448) -> (15.7814, 11.3916)
  line L500 (15.7814, 11.3916) -> (15.6509, 11.4162)
  line L501 (15.6509, 11.4162) -> (15.5187, 11.4184)
  line L502 (15.5187, 11.4184) -> (15.388, 11.3979)
  line L503 (15.388, 11.3979) -> (15.2619, 11.3543)
  line L504 (15.2619, 11.3543) -> (15.1433, 11.2873)
  line L505 (15.1433, 11.2873) -> (14.4806, 10.7591)
  line L506 (14.4806, 10.7591) -> (14.2878, 10.638)
  line L507 (14.2878, 10.638) -> (14.0874, 10.5359)
  line L508 (14.0874, 10.5359) -> (13.8809, 10.4527)
  line L509 (13.8809, 10.4527) -> (13.6692, 10.3882)
  line L510 (13.6692, 10.3882) -> (13.4537, 10.3425)
  line L511 (13.4537, 10.3425) -> (13.2356, 10.3152)
  line L512 (13.2356, 10.3152) -> (13.016, 10.3064)
  line L513 (13.016, 10.3064) -> (12.7962, 10.316)
  line L514 (12.7962, 10.316) -> (12.5775, 10.3439)
  line L515 (12.5775, 10.3439) -> (12.3609, 10.3898)
  line L516 (12.3609, 10.3898) -> (12.1478, 10.4539)
  line L517 (12.1478, 10.4539) -> (11.9394, 10.5358)
  line L518 (11.9394, 10.5358) -> (11.7368, 10.6356)
  line L519 (11.7368, 10.6356) -> (11.5413, 10.7531)
  line L520 (11.5413, 10.7531) -> (11.3541, 10.8882)
  line L521 (11.3541, 10.8882) -> (11.1764, 11.0408)
  line L522 (11.1764, 11.0408) -> (11.0239, 11.2185)
  line L523 (11.0239, 11.2185) -> (10.889, 11.4055)
  line L524 (10.889, 11.4055) -> (10.7716, 11.601)
  line L525 (10.7716, 11.601) -> (10.672, 11.8035)
  line L526 (10.672, 11.8035) -> (10.5901, 12.0119)
  line L527 (10.5901, 12.0119) -> (10.5262, 12.2249)
  line L528 (10.5262, 12.2249) -> (10.4803, 12.4414)
  line L529 (10.4803, 12.4414) -> (10.4525, 12.6601)
  line L530 (10.4525, 12.6601) -> (10.4429, 12.8799)
  line L531 (10.4429, 12.8799) -> (10.4516, 13.0994)
  line L532 (10.4516, 13.0994) -> (10.4788, 13.3175)
  line L533 (10.4788, 13.3175) -> (10.5246, 13.533)
  line L534 (10.5246, 13.533) -> (10.5889, 13.7447)
  line L535 (10.5889, 13.7447) -> (10.6721, 13.9513)
  line L536 (10.6721, 13.9513) -> (10.774, 14.1517)
  line L537 (10.774, 14.1517) -> (10.8949, 14.3446)
  line L538 (10.8949, 14.3446) -> (11.4231, 15.0073)
  line L539 (11.4231, 15.0073) -> (11.49, 15.1259)
  line L540 (11.49, 15.1259) -> (11.5336, 15.2521)
  line L541 (11.5336, 15.2521) -> (11.5541, 15.3828)
  line L542 (11.5541, 15.3828) -> (11.5519, 15.515)
  line L543 (11.5519, 15.515) -> (11.5273, 15.6455)
  line L544 (11.5273, 15.6455) -> (11.4806, 15.7713)
  line L545 (11.4806, 15.7713) -> (11.412, 15.8893)
  line L546 (11.412, 15.8893) -> (11.3688, 15.9407)
  line L547 (11.3688, 15.9407) -> (11.3688, 15.9408)
  line L548 (11.3688, 15.9408) -> (10.9534, 16.2488)
  line L549 (10.9534, 16.2488) -> (10.5098, 16.5147)
  line L550 (10.5098, 16.5147) -> (10.4916, 16.5205)
  line L551 (10.4916, 16.5205) -> (10.4457, 16.535)
  line L552 (10.4457, 16.535) -> (10.3104, 16.5532)
  line L553 (10.3104, 16.5532) -> (10.1762, 16.5482)
  line L554 (10.1762, 16.5482) -> (10.0462, 16.521)
  line L555 (10.0462, 16.521) -> (9.9232, 16.4725)
  line L556 (9.9232, 16.4725) -> (9.8104, 16.4035)
  line L557 (9.8104, 16.4035) -> (9.7105, 16.3149)
  line L558 (9.7105, 16.3149) -> (9.6267, 16.2077)
  line L559 (9.6267, 16.2077) -> (9.2165, 15.466)
  line L560 (9.2165, 15.466) -> (9.0847, 15.2804)
  line L561 (9.0847, 15.2804) -> (8.9387, 15.1094)
  line L562 (8.9387, 15.1094) -> (8.7798, 14.9534)
  line L563 (8.7798, 14.9534) -> (8.6089, 14.8129)
  line L564 (8.6089, 14.8129) -> (8.4273, 14.6881)
  line L565 (8.4273, 14.6881) -> (8.2362, 14.5794)
  line L566 (8.2362, 14.5794) -> (8.0367, 14.4872)
  line L567 (8.0367, 14.4872) -> (7.83, 14.412)
  line L568 (7.83, 14.412) -> (7.6173, 14.354)
  line L569 (7.6173, 14.354) -> (7.3996, 14.3136)
  line L570 (7.3996, 14.3136) -> (7.1782, 14.2912)
  line L571 (7.1782, 14.2912) -> (6.9543, 14.2871)
  line L572 (6.9543, 14.2871) -> (6.7289, 14.3018)
  line L573 (6.7289, 14.3018) -> (6.5034, 14.3355)
  line L574 (6.5034, 14.3355) -> (6.2787, 14.3887)
  line L575 (6.2787, 14.3887) -> (6.0562, 14.4618)
  line L576 (6.0562, 14.4618) -> (5.8474, 14.5675)
  line L577 (5.8474, 14.5675) -> (5.6511, 14.6888)
  line L578 (5.6511, 14.6888) -> (5.4679, 14.8245)
  line L579 (5.4679, 14.8245) -> (5.2983, 14.9734)
  line L580 (5.2983, 14.9734) -> (5.1429, 15.1346)
  line L581 (5.1429, 15.1346) -> (5.0023, 15.307)
  line L582 (5.0023, 15.307) -> (4.8771, 15.4894)
  line L583 (4.8771, 15.4894) -> (4.7677, 15.6809)
  line L584 (4.7677, 15.6809) -> (4.6748, 15.8802)
  line L585 (4.6748, 15.8802) -> (4.5988, 16.0864)
  line L586 (4.5988, 16.0864) -> (4.5405, 16.2983)
  line L587 (4.5405, 16.2983) -> (4.5003, 16.5149)
  line L588 (4.5003, 16.5149) -> (4.4787, 16.7351)
  line L589 (4.4787, 16.7351) -> (4.4765, 16.9578)
  line L590 (4.4765, 16.9578) -> (4.494, 17.1819)
  line L591 (4.494, 17.1819) -> (4.5319, 17.4064)
  line L592 (4.5319, 17.4064) -> (4.7662, 18.2208)
  line L593 (4.7662, 18.2208) -> (4.7826, 18.356)
  line L594 (4.7826, 18.356) -> (4.7746, 18.4893)
  line L595 (4.7746, 18.4893) -> (4.7436, 18.6179)
  line L596 (4.7436, 18.6179) -> (4.691, 18.7391)
  line L597 (4.691, 18.7391) -> (4.6183, 18.8503)
  line L598 (4.6183, 18.8503) -> (4.527, 18.9486)
  line L599 (4.527, 18.9486) -> (4.4184, 19.0314)
  line L600 (4.4184, 19.0314) -> (4.4015, 19.0402)
  line L601 (4.4015, 19.0402) -> (4.3588, 19.0624)
  line L602 (4.3588, 19.0624) -> (4.3588, 19.0624)
  line L603 (4.3588, 19.0624) -> (3.8571, 19.1881)
  line L604 (3.8571, 19.1881) -> (3.3455, 19.264)
  line L605 (3.3455, 19.264) -> (3.3266, 19.2624)
  line L606 (3.3266, 19.2624) -> (3.3265, 19.2624)
  line L607 (3.3265, 19.2624) -> (3.2786, 19.2582)
  line L608 (3.2786, 19.2582) -> (3.1466, 19.2232)
  line L609 (3.1466, 19.2232) -> (3.0245, 19.1673)
  line L610 (3.0245, 19.1673) -> (2.9148, 19.0924)
  line L611 (2.9148, 19.0924) -> (2.8198, 19.0005)
  line L612 (2.8198, 19.0005) -> (2.7419, 18.8936)
  line L613 (2.7419, 18.8936) -> (2.6835, 18.7735)
  line L614 (2.6835, 18.7735) -> (2.6471, 18.6423)
  line L615 (2.6471, 18.6423) -> (2.5519, 17.8002)
  line L616 (2.5519, 17.8002) -> (2.5012, 17.5783)
  line L617 (2.5012, 17.5783) -> (2.4317, 17.3644)
  line L618 (2.4317, 17.3644) -> (2.3445, 17.1595)
  line L619 (2.3445, 17.1595) -> (2.2404, 16.9643)
  line L620 (2.2404, 16.9643) -> (2.1204, 16.7795)
  line L621 (2.1204, 16.7795) -> (1.9854, 16.606)
  line L622 (1.9854, 16.606) -> (1.8363, 16.4445)
  line L623 (1.8363, 16.4445) -> (1.6742, 16.2959)
  line L624 (1.6742, 16.2959) -> (1.4998, 16.1609)
  line L625 (1.4998, 16.1609) -> (1.497, 16.1591)
  line L626 (1.497, 16.1591) -> (1.3963, 16.0937)
  line L627 (1.3963, 16.0937) -> (1.3142, 16.0403)
  line L628 (1.3142, 16.0403) -> (1.1182, 15.9349)
  line L629 (1.1182, 15.9349) -> (0.9129, 15.8454)
  line L630 (0.9129, 15.8454) -> (0.6991, 15.7727)
  line L631 (0.6991, 15.7727) -> (0.4778, 15.7176)
  line L632 (0.4778, 15.7176) -> (0.2499, 15.6808)
  line L633 (0.2499, 15.6808) -> (0.2354, 15.6797)
  line L634 (0.2354, 15.6797) -> (0.1396, 15.6724)
  line L635 (0.1396, 15.6724) -> (0.0163, 15.6631)
  line L636 (0.0163, 15.6631) -> (-0.2171, 15.6809)
  line L637 (-0.2171, 15.6809) -> (-0.4449, 15.7178)
  line L638 (-0.4449, 15.7178) -> (-0.666, 15.773)
  line L639 (-0.666, 15.773) -> (-0.8797, 15.8458)
  line L640 (-0.8797, 15.8458) -> (-1.0849, 15.9352)
  line L641 (-1.0849, 15.9352) -> (-1.1695, 15.9807)
  line L642 (-1.1695, 15.9807) -> (-1.265, 16.0322)
  line L643 (-1.265, 16.0322) -> (-1.2808, 16.0407)
  line L644 (-1.2808, 16.0407) -> (-1.3628, 16.094)
  line L645 (-1.3628, 16.094) -> (-1.464, 16.1598)
  line L646 (-1.464, 16.1598) -> (-1.4664, 16.1613)
  line L647 (-1.4664, 16.1613) -> (-1.6407, 16.2963)
  line L648 (-1.6407, 16.2963) -> (-1.8029, 16.4448)
  line L649 (-1.8029, 16.4448) -> (-1.9519, 16.6062)
  line L650 (-1.9519, 16.6062) -> (-2.087, 16.7797)
  line L651 (-2.087, 16.7797) -> (-2.207, 16.9644)
  line L652 (-2.207, 16.9644) -> (-2.3112, 17.1596)
  line L653 (-2.3112, 17.1596) -> (-2.3985, 17.3645)
  line L654 (-2.3985, 17.3645) -> (-2.4681, 17.5782)
  line L655 (-2.4681, 17.5782) -> (-2.519, 17.8001)
  line L656 (-2.519, 17.8001) -> (-2.6142, 18.6422)
  line L657 (-2.6142, 18.6422) -> (-2.6507, 18.7734)
  line L658 (-2.6507, 18.7734) -> (-2.7091, 18.8935)
  line L659 (-2.7091, 18.8935) -> (-2.787, 19.0004)
  line L660 (-2.787, 19.0004) -> (-2.882, 19.0923)
  line L661 (-2.882, 19.0923) -> (-2.9917, 19.1672)
  line L662 (-2.9917, 19.1672) -> (-3.1137, 19.2231)
  line L663 (-3.1137, 19.2231) -> (-3.2456, 19.2581)
  line L664 (-3.2456, 19.2581) -> (-3.2646, 19.2597)
  line L665 (-3.2646, 19.2597) -> (-3.3126, 19.2639)
  line L666 (-3.3126, 19.2639) -> (-3.3126, 19.2639)
  line L667 (-3.3126, 19.2639) -> (-3.8295, 19.2483)
  line L668 (-3.8295, 19.2483) -> (-4.3425, 19.1821)
  line L669 (-4.3425, 19.1821) -> (-4.3594, 19.1733)
  line L670 (-4.3594, 19.1733) -> (-4.3594, 19.1733)
  line L671 (-4.3594, 19.1733) -> (-4.4021, 19.1511)
  line L672 (-4.4021, 19.1511) -> (-4.5107, 19.0683)
  line L673 (-4.5107, 19.0683) -> (-4.602, 18.9699)
  line L674 (-4.602, 18.9699) -> (-4.6748, 18.8588)
  line L675 (-4.6748, 18.8588) -> (-4.7274, 18.7375)
  line L676 (-4.7274, 18.7375) -> (-4.7584, 18.6089)
  line L677 (-4.7584, 18.6089) -> (-4.7664, 18.4757)
  line L678 (-4.7664, 18.4757) -> (-4.7498, 18.3405)
  line L679 (-4.7498, 18.3405) -> (-4.5156, 17.5261)
  line L680 (-4.5156, 17.5261) -> (-4.4775, 17.3016)
  line L681 (-4.4775, 17.3016) -> (-4.4598, 17.0775)
  line L682 (-4.4598, 17.0775) -> (-4.4619, 16.8548)
  line L683 (-4.4619, 16.8548) -> (-4.4834, 16.6346)
  line L684 (-4.4834, 16.6346) -> (-4.5235, 16.4179)
  line L685 (-4.5235, 16.4179) -> (-4.5819, 16.206)
  line L686 (-4.5819, 16.206) -> (-4.6578, 15.9998)
  line L687 (-4.6578, 15.9998) -> (-4.7507, 15.8004)
  line L688 (-4.7507, 15.8004) -> (-4.8602, 15.6089)
  line L689 (-4.8602, 15.6089) -> (-4.9855, 15.4265)
  line L690 (-4.9855, 15.4265) -> (-5.1262, 15.2541)
  line L691 (-5.1262, 15.2541) -> (-5.2817, 15.0929)
  line L692 (-5.2817, 15.0929) -> (-5.4514, 14.9439)
  line L693 (-5.4514, 14.9439) -> (-5.6348, 14.8083)
  line L694 (-5.6348, 14.8083) -> (-5.8312, 14.6871)
  line L695 (-5.8312, 14.6871) -> (-6.0402, 14.5813)
  line L696 (-6.0402, 14.5813) -> (-6.2627, 14.5085)
  line L697 (-6.2627, 14.5085) -> (-6.4872, 14.4554)
  line L698 (-6.4872, 14.4554) -> (-6.7127, 14.4218)
  line L699 (-6.7127, 14.4218) -> (-6.938, 14.4072)
  line L700 (-6.938, 14.4072) -> (-7.1618, 14.4113)
  line L701 (-7.1618, 14.4113) -> (-7.3831, 14.4338)
  line L702 (-7.3831, 14.4338) -> (-7.6007, 14.4742)
  line L703 (-7.6007, 14.4742) -> (-7.8134, 14.5322)
  line L704 (-7.8134, 14.5322) -> (-8.02, 14.6075)
  line L705 (-8.02, 14.6075) -> (-8.2195, 14.6996)
  line L706 (-8.2195, 14.6996) -> (-8.4106, 14.8082)
  line L707 (-8.4106, 14.8082) -> (-8.5922, 14.9329)
  line L708 (-8.5922, 14.9329) -> (-8.7632, 15.0734)
  line L709 (-8.7632, 15.0734) -> (-8.9222, 15.2292)
  line L710 (-8.9222, 15.2292) -> (-9.0683, 15.4001)
  line L711 (-9.0683, 15.4001) -> (-9.2002, 15.5856)
  line L712 (-9.2002, 15.5856) -> (-9.6105, 16.3272)
  line L713 (-9.6105, 16.3272) -> (-9.6944, 16.4344)
  line L714 (-9.6944, 16.4344) -> (-9.7943, 16.523)
  line L715 (-9.7943, 16.523) -> (-9.9072, 16.592)
  line L716 (-9.9072, 16.592) -> (-10.0301, 16.6405)
  line L717 (-10.0301, 16.6405) -> (-10.1601, 16.6677)
  line L718 (-10.1601, 16.6677) -> (-10.2942, 16.6727)
  line L719 (-10.2942, 16.6727) -> (-10.4295, 16.6545)
  line L720 (-10.4295, 16.6545) -> (-10.4477, 16.6487)
  line L721 (-10.4477, 16.6487) -> (-10.4935, 16.6342)
  line L722 (-10.4935, 16.6342) -> (-10.4936, 16.6342)
  line L723 (-10.4936, 16.6342) -> (-10.9372, 16.3683)
  line L724 (-10.9372, 16.3683) -> (-11.3526, 16.0603)
  line L725 (-11.3526, 16.0603) -> (-11.3526, 16.0602)
  line L726 (-11.3526, 16.0602) -> (-11.3958, 16.0088)
  line L727 (-11.3958, 16.0088) -> (-11.4644, 15.8907)
  line L728 (-11.4644, 15.8907) -> (-11.5112, 15.7649)
  line L729 (-11.5112, 15.7649) -> (-11.5358, 15.6344)
  line L730 (-11.5358, 15.6344) -> (-11.538, 15.5022)
  line L731 (-11.538, 15.5022) -> (-11.5175, 15.3715)
  line L732 (-11.5175, 15.3715) -> (-11.4739, 15.2454)
  line L733 (-11.4739, 15.2454) -> (-11.4069, 15.1268)
  line L734 (-11.4069, 15.1268) -> (-10.8787, 14.4641)
  line L735 (-10.8787, 14.4641) -> (-10.7576, 14.2713)
  line L736 (-10.7576, 14.2713) -> (-10.6555, 14.0709)
  line L737 (-10.6555, 14.0709) -> (-10.5723, 13.8644)
  line L738 (-10.5723, 13.8644) -> (-10.5078, 13.6527)
  line L739 (-10.5078, 13.6527) -> (-10.4621, 13.4372)
  line L740 (-10.4621, 13.4372) -> (-10.4348, 13.2191)
  line L741 (-10.4348, 13.2191) -> (-10.426, 12.9995)
  line L742 (-10.426, 12.9995) -> (-10.4356, 12.7797)
  line L743 (-10.4356, 12.7797) -> (-10.4635, 12.561)
  line L744 (-10.4635, 12.561) -> (-10.5094, 12.3444)
  line L745 (-10.5094, 12.3444) -> (-10.5735, 12.1313)
  line L746 (-10.5735, 12.1313) -> (-10.6554, 11.9229)
  line L747 (-10.6554, 11.9229) -> (-10.7552, 11.7203)
  line L748 (-10.7552, 11.7203) -> (-10.8727, 11.5248)
  line L749 (-10.8727, 11.5248) -> (-11.0078, 11.3376)
  line L750 (-11.0078, 11.3376) -> (-11.1604, 11.16)
  line L751 (-11.1604, 11.16) -> (-11.3381, 11.0074)
  line L752 (-11.3381, 11.0074) -> (-11.5252, 10.8725)
  line L753 (-11.5252, 10.8725) -> (-11.7207, 10.7551)
  line L754 (-11.7207, 10.7551) -> (-11.9232, 10.6555)
  line L755 (-11.9232, 10.6555) -> (-12.1316, 10.5736)
  line L756 (-12.1316, 10.5736) -> (-12.3446, 10.5097)
  line L757 (-12.3446, 10.5097) -> (-12.5611, 10.4638)
  line L758 (-12.5611, 10.4638) -> (-12.7798, 10.436)
  line L759 (-12.7798, 10.436) -> (-12.9996, 10.4264)
  line L760 (-12.9996, 10.4264) -> (-13.2191, 10.4351)
  line L761 (-13.2191, 10.4351) -> (-13.4372, 10.4623)
  line L762 (-13.4372, 10.4623) -> (-13.6527, 10.5081)
  line L763 (-13.6527, 10.5081) -> (-13.8644, 10.5724)
  line L764 (-13.8644, 10.5724) -> (-14.071, 10.6556)
  line L765 (-14.071, 10.6556) -> (-14.2714, 10.7575)
  line L766 (-14.2714, 10.7575) -> (-14.4643, 10.8784)
  line L767 (-14.4643, 10.8784) -> (-15.127, 11.4066)
  line L768 (-15.127, 11.4066) -> (-15.2456, 11.4735)
  line L769 (-15.2456, 11.4735) -> (-15.3718, 11.5171)
  line L770 (-15.3718, 11.5171) -> (-15.5025, 11.5376)
  line L771 (-15.5025, 11.5376) -> (-15.6347, 11.5354)
  line L772 (-15.6347, 11.5354) -> (-15.7652, 11.5108)
  line L773 (-15.7652, 11.5108) -> (-15.891, 11.4641)
  line L774 (-15.891, 11.4641) -> (-16.009, 11.3955)
  line L775 (-16.009, 11.3955) -> (-16.0236, 11.3833)
  line L776 (-16.0236, 11.3833) -> (-16.0604, 11.3523)
  line L777 (-16.0604, 11.3523) -> (-16.0605, 11.3523)
  line L778 (-16.0605, 11.3523) -> (-16.3685, 10.9369)
  line L779 (-16.3685, 10.9369) -> (-16.6344, 10.4933)
  line L780 (-16.6344, 10.4933) -> (-16.6344, 10.4932)
  line L781 (-16.6344, 10.4932) -> (-16.6547, 10.4292)
  line L782 (-16.6547, 10.4292) -> (-16.6729, 10.2939)
  line L783 (-16.6729, 10.2939) -> (-16.6679, 10.1597)
  line L784 (-16.6679, 10.1597) -> (-16.6407, 10.0297)
  line L785 (-16.6407, 10.0297) -> (-16.5921, 9.9068)
  line L786 (-16.5921, 9.9068) -> (-16.5231, 9.7939)
  line L787 (-16.5231, 9.7939) -> (-16.4345, 9.694)
  line L788 (-16.4345, 9.694) -> (-16.3273, 9.6102)
  line L789 (-16.3273, 9.6102) -> (-15.5857, 9.2)
  line L790 (-15.5857, 9.2) -> (-15.4001, 9.0682)
  line L791 (-15.4001, 9.0682) -> (-15.2291, 8.9223)
  line L792 (-15.2291, 8.9223) -> (-15.0731, 8.7633)
  line L793 (-15.0731, 8.7633) -> (-14.9325, 8.5924)
  line L794 (-14.9325, 8.5924) -> (-14.8077, 8.4108)
  line L795 (-14.8077, 8.4108) -> (-14.699, 8.2197)
  line L796 (-14.699, 8.2197) -> (-14.6069, 8.0202)
  line L797 (-14.6069, 8.0202) -> (-14.5317, 7.8135)
  line L798 (-14.5317, 7.8135) -> (-14.4737, 7.6008)
  line L799 (-14.4737, 7.6008) -> (-14.4333, 7.3831)
  line L800 (-14.4333, 7.3831) -> (-14.4109, 7.1617)
  line L801 (-14.4109, 7.1617) -> (-14.4068, 6.9378)
  line L802 (-14.4068, 6.9378) -> (-14.4215, 6.7125)
  line L803 (-14.4215, 6.7125) -> (-14.4552, 6.4869)
  line L804 (-14.4552, 6.4869) -> (-14.5084, 6.2623)
  line L805 (-14.5084, 6.2623) -> (-14.5815, 6.0397)
  line L806 (-14.5815, 6.0397) -> (-14.6872, 5.8309)
  line L807 (-14.6872, 5.8309) -> (-14.8085, 5.6346)
  line L808 (-14.8085, 5.6346) -> (-14.9442, 5.4514)
  line L809 (-14.9442, 5.4514) -> (-15.0931, 5.2818)
  line L810 (-15.0931, 5.2818) -> (-15.2543, 5.1264)
  line L811 (-15.2543, 5.1264) -> (-15.4267, 4.9858)
  line L812 (-15.4267, 4.9858) -> (-15.6091, 4.8606)
  line L813 (-15.6091, 4.8606) -> (-15.8006, 4.7512)
  line L814 (-15.8006, 4.7512) -> (-15.9999, 4.6583)
  line L815 (-15.9999, 4.6583) -> (-16.2061, 4.5823)
  line L816 (-16.2061, 4.5823) -> (-16.418, 4.524)
  line L817 (-16.418, 4.524) -> (-16.6346, 4.4838)
  line L818 (-16.6346, 4.4838) -> (-16.8548, 4.4622)
  line L819 (-16.8548, 4.4622) -> (-17.0775, 4.46)
  line L820 (-17.0775, 4.46) -> (-17.3016, 4.4775)
  line L821 (-17.3016, 4.4775) -> (-17.5261, 4.5154)
  line L822 (-17.5261, 4.5154) -> (-18.3405, 4.7497)
  line L823 (-18.3405, 4.7497) -> (-18.4757, 4.7661)
  line L824 (-18.4757, 4.7661) -> (-18.609, 4.7581)
  line L825 (-18.609, 4.7581) -> (-18.7376, 4.7271)
  line L826 (-18.7376, 4.7271) -> (-18.8588, 4.6745)
  line L827 (-18.8588, 4.6745) -> (-18.97, 4.6018)
  line L828 (-18.97, 4.6018) -> (-19.0683, 4.5105)
  line L829 (-19.0683, 4.5105) -> (-19.1511, 4.402)
  line L830 (-19.1511, 4.402) -> (-19.1821, 4.3424)
  line L831 (-19.1821, 4.3424) -> (-19.1821, 4.3423)
  line L832 (-19.1821, 4.3423) -> (-19.3078, 3.8406)
  line L833 (-19.3078, 3.8406) -> (-19.3837, 3.3291)
  line L834 (-19.3837, 3.3291) -> (-19.3837, 3.329)
  line L835 (-19.3837, 3.329) -> (-19.3779, 3.2621)
  line L836 (-19.3779, 3.2621) -> (-19.3429, 3.1301)
  line L837 (-19.3429, 3.1301) -> (-19.287, 3.008)
  line L838 (-19.287, 3.008) -> (-19.2121, 2.8983)
  line L839 (-19.2121, 2.8983) -> (-19.1202, 2.8033)
  line L840 (-19.1202, 2.8033) -> (-19.0133, 2.7254)
  line L841 (-19.0133, 2.7254) -> (-18.8932, 2.667)
  line L842 (-18.8932, 2.667) -> (-18.762, 2.6306)
  line L843 (-18.762, 2.6306) -> (-17.9199, 2.5354)
  line L844 (-17.9199, 2.5354) -> (-17.698, 2.4847)
  line L845 (-17.698, 2.4847) -> (-17.4841, 2.4152)
  line L846 (-17.4841, 2.4152) -> (-17.2792, 2.328)
  line L847 (-17.2792, 2.328) -> (-17.084, 2.2239)
  line L848 (-17.084, 2.2239) -> (-16.8992, 2.1039)
  line L849 (-16.8992, 2.1039) -> (-16.7257, 1.9689)
  line L850 (-16.7257, 1.9689) -> (-16.5642, 1.8198)
  line L851 (-16.5642, 1.8198) -> (-16.4156, 1.6577)
  line L852 (-16.4156, 1.6577) -> (-16.2806, 1.4833)
  line L853 (-16.2806, 1.4833) -> (-16.2788, 1.4805)
  line L854 (-16.2788, 1.4805) -> (-16.2134, 1.3798)
  line L855 (-16.2134, 1.3798) -> (-16.16, 1.2977)
  line L856 (-16.16, 1.2977) -> (-16.0546, 1.1017)
  line L857 (-16.0546, 1.1017) -> (-15.9651, 0.8964)
  line L858 (-15.9651, 0.8964) -> (-15.8924, 0.6826)
  line L859 (-15.8924, 0.6826) -> (-15.8373, 0.4613)
  line L860 (-15.8373, 0.4613) -> (-15.8005, 0.2334)
  line L861 (-15.8005, 0.2334) -> (-15.7994, 0.2189)
  line L862 (-15.7994, 0.2189) -> (-15.7921, 0.1231)
  line L863 (-15.7921, 0.1231) -> (-15.7828, -0.0002)
  line L864 (-15.7828, -0.0002) -> (-15.8006, -0.2336)
  line L865 (-15.8006, -0.2336) -> (-15.8375, -0.4614)
  line L866 (-15.8375, -0.4614) -> (-15.8927, -0.6825)
  line L867 (-15.8927, -0.6825) -> (-15.9655, -0.8962)
  line L868 (-15.9655, -0.8962) -> (-16.0549, -1.1014)
  line L869 (-16.0549, -1.1014) -> (-16.1004, -1.186)
  line L870 (-16.1004, -1.186) -> (-16.1519, -1.2815)
  line L871 (-16.1519, -1.2815) -> (-16.1604, -1.2973)
  line L872 (-16.1604, -1.2973) -> (-16.2137, -1.3793)
  line L873 (-16.2137, -1.3793) -> (-16.2795, -1.4805)
  line L874 (-16.2795, -1.4805) -> (-16.281, -1.4829)
  line L875 (-16.281, -1.4829) -> (-16.4159, -1.6572)
  line L876 (-16.4159, -1.6572) -> (-16.5645, -1.8194)
  line L877 (-16.5645, -1.8194) -> (-16.7259, -1.9684)
  line L878 (-16.7259, -1.9684) -> (-16.8994, -2.1035)
  line L879 (-16.8994, -2.1035) -> (-17.0841, -2.2235)
  line L880 (-17.0841, -2.2235) -> (-17.2793, -2.3277)
  line L881 (-17.2793, -2.3277) -> (-17.4842, -2.415)
  line L882 (-17.4842, -2.415) -> (-17.6979, -2.4846)
  line L883 (-17.6979, -2.4846) -> (-17.9198, -2.5355)
  line L884 (-17.9198, -2.5355) -> (-18.7619, -2.6307)
  line L885 (-18.7619, -2.6307) -> (-18.8931, -2.6672)
  line L886 (-18.8931, -2.6672) -> (-19.0132, -2.7256)
  line L887 (-19.0132, -2.7256) -> (-19.1201, -2.8035)
  line L888 (-19.1201, -2.8035) -> (-19.212, -2.8985)
  line L889 (-19.212, -2.8985) -> (-19.2869, -3.0082)
  line L890 (-19.2869, -3.0082) -> (-19.3428, -3.1302)
  line L891 (-19.3428, -3.1302) -> (-19.3778, -3.2621)
  line L892 (-19.3778, -3.2621) -> (-19.3836, -3.3291)
  line L893 (-19.3836, -3.3291) -> (-19.3836, -3.3292)
  constraints: 1788 end point, 421 perpendicular, 241 parallel
extrude "Extrusion1" add sketch "Sketch1" along normal blind 30
sketch "Sketch2" plane through (0, 30, 0) normal (0, 1, 0) x (1, 0, 0)
  circle A0 centre (0, 0) radius 20
  dimension "d2" = 40
  constraints: 1 centre point, 1 coincident
  measures "d2" diameter of A0
ref_plane "Work Plane1" through (0, 31.5, 0) normal (0, 1, 0) x (1, 0, 0)
sketch "Sketch3" plane through (0, 31.5, 0) normal (0, 1, 0) x (1, 0, 0)
  circle A0 centre (0, 0) radius 21
  dimension "d4" = 42
  constraints: 1 centre point, 1 coincident
  measures "d4" diameter of A0
loft "Loft1" add profiles "Sketch2", "Sketch3"
sketch "Sketch4" plane through (0, 0, 0) normal (0, -1, 0) x (1, 0, 0)
  circle A0 centre (0, 0) radius 20
  dimension "d9" = 40
  constraints: 1 centre point, 1 coincident
  measures "d9" diameter of A0
ref_plane "Work Plane2" through (0, -1.5, 0) normal (0, -1, 0) x (1, 0, 0)
sketch "Sketch5" plane through (0, -1.5, 0) normal (0, -1, 0) x (1, 0, 0)
  circle A0 centre (0, 0) radius 21
  dimension "d11" = 42
  constraints: 1 centre point, 1 coincident
  measures "d11" diameter of A0
loft "Loft2" add profiles "Sketch4", "Sketch5"
sketch "Sketch6" plane through (0, -1.5, 0) normal (0, -1, 0) x (1, 0, 0)
  point P0 (0, 0)
  point P1 (0, 0)
  constraints: 1 coincident
hole "Hole1" at (0, -1.5, 0) direction (0, 1, 0) diameter 6.28 end through all counterbore diameter 15 counterbore depth 7